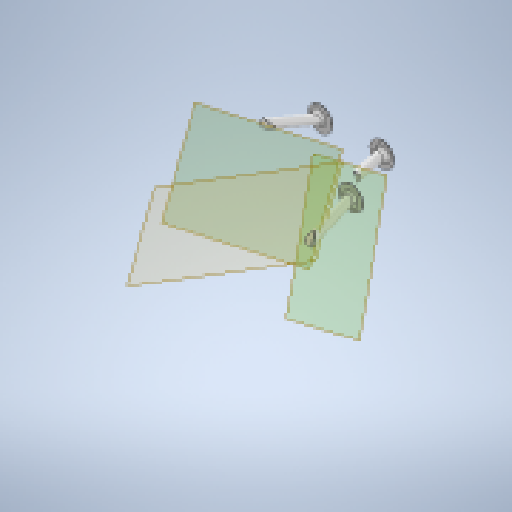
# Autodesk Inventor part: Brazos
Saved by Autodesk Inventor 2024 (Build 280153000, 153)
## iProperties
Created: 2024-07-14
Part Number: Brazos
Material: Genérico
Document SubType Name: Modeling
Designer: sergi
Density: 1 g/cm^3
Appearance: Valor por defecto
Author: sergi
Autodesk Inventor part; units mm, degrees
sketch "Boceto1" plane through (0, 0, 0) normal (0, 0, 1) x (1, 0, 0)
  arc A0 (-25.980762, -64.848267) -> (25.980762, -64.848267) centre (0, -49.848267) ccw
  line L0 (69.019238, 9.69656) -> (25.980762, -64.848267)
  arc A1 (69.019238, 9.69656) -> (43.038476, 54.69656) centre (43.038476, 24.69656) ccw
  line L1 (-43.038476, 54.69656) -> (43.038476, 54.69656)
  arc A2 (-43.038476, 54.69656) -> (-69.019238, 9.69656) centre (-43.038476, 24.69656) ccw
  line L2 (-25.980762, -64.848267) -> (-69.019238, 9.69656)
  line L3 (0, -49.848267) -> (0, -59.848267)
  circle A3 centre (0, -59.848267) radius 7.5
  point P0 (0, 0)
  dimension "d2" = 10
  dimension "d3" = 15
  constraints: 2 coincident, 2 end point, 1 centre point, 1 vertical
  measures "d2" distance of L3.start L3.end
  measures "d3" diameter of A3
ref_plane "Plano de trabajo1" through (-0.019887, -110.372572, 72.1) normal (1, 0, -0.0000689) x (-0.0000246, 0.9341866, -0.3567849)
sketch "Boceto2" plane through (-0.019887, -110.372572, 72.1) normal (1, 0, -0.0000689) x (-0.0000246, 0.9341866, -0.3567849)
  ellipse E0 centre (82.265185, -45.76069) end of major axis (89.271584, -43.084803) minor radius 0.000517
  line L0 (59, 95.445569) -> (-36.467526, 58.987261)
  line L1 (154.467526, 58.987261) -> (59, 95.445569)
  line L2 (118, 0) -> (154.467526, 58.987261)
  line L3 (118, 0) -> (0, 0)
  line L4 (0, 0) -> (-36.467526, 58.987261)
  ellipse E1 centre (82.265185, -45.76069) end of major axis (54.239588, -56.464237) minor radius 0.002067 (68.253025, -51.114136) -> (68.251748, -51.110791) ccw
  line L5 (68.253025, -51.114136) -> (137.892858, -24.520436)
  ellipse E2 centre (82.265185, -45.76069) end of major axis (54.239588, -56.464237) minor radius 0.002067 (68.253025, -51.114136) -> (68.251748, -51.110791) ccw
  ellipse E3 centre (82.265185, -45.76069) end of major axis (54.239588, -56.464237) minor radius 0.002067 (68.253025, -51.114136) -> (68.251748, -51.110791) ccw
  line L6 (54.239598, -56.464235) -> (0, 0)
  line L7 (82.265185, -45.76069) -> (38.307423, 0)
  ellipse E4 centre (72.923319, -49.328539) end of major axis (79.929718, -46.652652) minor radius 0.000517
  line L8 (72.923319, -49.328539) -> (13.250704, 12.791548)
  point P0 (128.832765, -27.97558)
  constraints: 6 end point, 2 parallel, 1 point on line, 3 other
sweep "Barrido1" add profiles "Boceto1" path "Boceto2" path curves L8 contours A3
ref_plane "Plano de trabajo2" through (-0.019887, -110.372572, 72.1) normal (-0.5257124, -0.3035156, -0.7946727) x (0.0000246, -0.9341866, 0.3567849)
ref_plane "Plano de trabajo3" through (71.579739, -47.983878, 95.634962) normal (0.5256763, -0.3034994, -0.7947028) x (-0.2628994, 0.830501, -0.4910723)
split body "Dividir1" result two bodies by plane through (71.579739, -47.983878, 95.634962) normal (0.5256763, -0.3034994, -0.7947028) first body at (6.955897, -74.969081, 37.610548)
split body "Dividir2" result two bodies by plane through (-0.019887, -110.372572, 72.1) normal (-0.5257124, -0.3035156, -0.7946727) bodies 2 first body at (6.912454, -73.047786, 28.55912)
split body "Dividir3" result two bodies by plane through (-0.019887, -110.372572, 72.1) normal (-0.5257124, -0.3035156, -0.7946727) bodies 3 first body at (-5.42219, -92.704981, 67.231243)
combine bodies "Combinar1" operation type add bodies to combine 4 6 5
sketch "Boceto3" plane through (0, -59.848267, 0) normal (0, 0, -1) x (-1, 0, 0)
  circle A0 centre (0, 0) radius 20
  point P0 (0, 59.848267)
  dimension "d9" = 40
  constraints: 1 centre point
  measures "d9" diameter of A0
extrude "Extrusión1" add sketch "Boceto3" along normal blind 1 bodies 4
fillet "Empalme1" radius 5 1 edges at (-7.5, -59.8483, 0)
sketch "Boceto4" plane through (-0.019887, -110.372572, 72.1) normal (1, 0, -0.0000689) x (-0.0000246, 0.9341866, -0.3567849)
  ellipse E0 centre (25.523521, 0.015362) end of major axis (14.998906, 2.312406) minor radius 4.120837 (35.115083, 0) -> (15.961471, 0) ccw
  ellipse E1 centre (25.553031, -0.015359) end of major axis (36.077552, -2.311708) minor radius 4.120133 (35.115083, 0) -> (15.961471, 0) ccw
  ellipse E2 centre (13.250704, 12.791548) end of major axis (20.257103, 15.467435) minor radius 0.000517
  ellipse E3 centre (25.553031, -0.015359) end of major axis (36.077552, -2.311708) minor radius 4.120133 (35.115083, 0) -> (15.961471, 0) ccw
  ellipse E4 centre (25.523521, 0.015362) end of major axis (14.998906, 2.312406) minor radius 4.120837 (35.115083, 0) -> (15.961471, 0) ccw
  line L0 (-5, -26) -> (79, -26)
  line L1 (79, -26) -> (79, 56)
  line L2 (79, 56) -> (-5, 56)
  line L3 (-5, 56) -> (-5, -26)
  line L4 (15.961471, 0) -> (79, 0)
  point P0 (128.832765, -27.97558)
  constraints: 10 end point, 2 parallel, 1 horizontal, 1 perpendicular, 1 point on line, 5 other
ref_plane "Plano de trabajo4" through (-0.02028, -95.461581, 66.405188) normal (-0.0030519, -0.9208692, -0.3898597) x (0.9999945, -0.0033141, 0)
sketch "Boceto5" plane through (-0.02028, -95.461581, 66.405188) normal (-0.0030519, -0.9208692, -0.3898597) x (0.9999945, -0.0033141, 0)
  ellipse E0 centre (0.019013, 11.102778) end of major axis (7.519013, 11.102778) minor radius 2.923948
  ellipse E1 centre (-0.005058, -6.6557) end of major axis (6.539295, -15.49658) minor radius 4.535858 (0, 0) -> (-0.059771, -13.268736) ccw
  ellipse E2 centre (-0.005001, -6.613101) end of major axis (6.577576, 2.215151) minor radius 4.506259 (-0.059771, -13.268736) -> (0, 0) ccw
  line L0 (-14, 35.791605) -> (14.4744, 35.791605)
  line L1 (14.4744, 35.791605) -> (14.4744, 0)
  line L2 (14.4744, 0) -> (-14, 0)
  line L3 (-14, 0) -> (-14, 35.791605)
  point P0 (-0.296092, -98.367276)
  point P1 (-7.491076, 0)
  point P2 (7.501189, 0)
  constraints: 8 end point, 2 parallel, 1 horizontal, 1 perpendicular, 2 other
sweep "Barrido2" cut profiles "Boceto5" path "Boceto4" bodies 7 path curves L4 contours E0 | E1 L2 L3 L0 L1 E2
pattern_circular "Patrón circular1" count 3 over 360 about axis through (0, 0, -10) along (0, 0, 1) bodies 4
